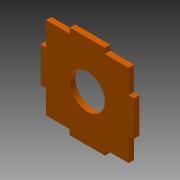
# Autodesk Inventor part: Top
Saved by Autodesk Inventor 2014 (Build 180170000, 170)
## iProperties
Created: 2014-11-21
Part Number: Top
Material: Generic
Document SubType Name: Modeling
Designer: JLM
Density: 1 g/cm^3
Appearance: Default
Author: JLM
Autodesk Inventor part; units mm, degrees
ref_plane "YZ Plane" through (0, 0, 0) normal (1, 0, 0) x (0, 1, 0)
ref_plane "XZ Plane" through (0, 0, 0) normal (0, 1, 0) x (-1, 0, 0)
ref_plane "XY Plane" through (0, 0, 0) normal (0, 0, 1) x (1, 0, 0)
sketch "Sketch1" plane through (0, 0, 0) normal (0, 0, 1) x (1, 0, 0)
  line L0 (-25.4, -25.4) -> (25.4, -25.4)
  line L1 (25.4, -25.4) -> (25.4, 25.4)
  line L2 (25.4, 25.4) -> (-25.4, 25.4)
  line L3 (-25.4, 25.4) -> (-25.4, -25.4)
  line L4 (-25.4, -25.4) -> (25.4, 25.4) construction
  line L5 (25.4, -25.4) -> (-25.4, 25.4) construction
  point P0 (0, 0)
  dimension "d0" = 50.8
  dimension "d1" = 50.8
  constraints: 12 end point, 2 midpoint, 2 parallel, 1 horizontal, 1 perpendicular
  measures "d0" distance of L2.end L1.end
  measures "d1" distance of L1.end L0.end
extrude "Extrusion1" add sketch "Sketch1" against normal blind 2.921
sketch "Sketch2" plane through (0, 0, 0) normal (0, 0, 1) x (1, 0, 0)
  line L0 (-25.4, 25.4) -> (-9.525, 25.4)
  line L1 (-9.525, 25.4) -> (-9.525, 22.479)
  line L2 (-9.525, 22.479) -> (-22.479, 22.479)
  line L3 (-25.4, 22.479) -> (-25.4, 25.4)
  line L4 (-25.4, 25.4) -> (-22.225, 25.4)
  line L5 (-22.479, 22.479) -> (-22.479, 9.525)
  line L6 (-22.479, 9.525) -> (-25.4, 9.525)
  line L7 (-25.4, 9.525) -> (-25.4, 25.4)
  line L8 (25.4, 25.4) -> (-25.4, 25.4) projected
  line L9 (-25.4, 25.4) -> (-25.4, -25.4) projected
  line L10 (0, 4.0972) -> (0, 8.5289)
  line L11 (-5.3828, 0) -> (-2.3228, 0)
  line L12 (25.4, 25.4) -> (9.525, 25.4)
  line L13 (9.525, 25.4) -> (9.525, 22.479)
  line L14 (9.525, 22.479) -> (22.479, 22.479)
  line L15 (25.4, 22.479) -> (25.4, 25.4)
  line L16 (25.4, 25.4) -> (22.225, 25.4)
  line L17 (22.479, 22.479) -> (22.479, 9.525)
  line L18 (22.479, 9.525) -> (25.4, 9.525)
  line L19 (25.4, 9.525) -> (25.4, 25.4)
  line L20 (-25.4, -25.4) -> (-9.525, -25.4)
  line L21 (-9.525, -25.4) -> (-9.525, -22.479)
  line L22 (-9.525, -22.479) -> (-22.479, -22.479)
  line L23 (-25.4, -22.479) -> (-25.4, -25.4)
  line L24 (-25.4, -25.4) -> (-22.225, -25.4)
  line L25 (-22.479, -22.479) -> (-22.479, -9.525)
  line L26 (-22.479, -9.525) -> (-25.4, -9.525)
  line L27 (-25.4, -9.525) -> (-25.4, -25.4)
  line L28 (25.4, -25.4) -> (-25.4, -25.4)
  line L29 (25.4, -25.4) -> (9.525, -25.4)
  line L30 (9.525, -25.4) -> (9.525, -22.479)
  line L31 (9.525, -22.479) -> (22.479, -22.479)
  line L32 (25.4, -22.479) -> (25.4, -25.4)
  line L33 (25.4, -25.4) -> (22.225, -25.4)
  line L34 (22.479, -22.479) -> (22.479, -9.525)
  line L35 (22.479, -9.525) -> (25.4, -9.525)
  line L36 (25.4, -9.525) -> (25.4, -25.4)
  point P0 (0, -8.5289)
  dimension "d59" = 2.921
  dimension "d61" = 15.875
  dimension "d62" = 2.921
  constraints: 70 end point, 29 symmetric about line, 5 parallel, 3 perpendicular, 2 collinear, 2 horizontal
  measures "d59" distance of L0.end L1.end
  measures "d61" distance of L1.end L3.start
  measures "d62" distance of L5.end L6.end
hole "Hole1" at (0, 0, 0) direction (0, 0, -1) diameter 19.05 end through all
extrude "Extrusion3" cut sketch "Sketch2" against normal up to next
equation "\"d1\" = d0"
equation "\"d62\" = d59"
equation "\"d53\" = 0.5 * d0"
body "Solid1"
